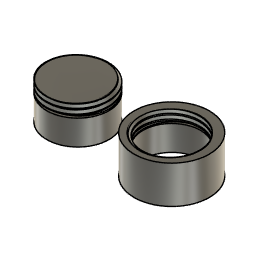
Threads Test (Autodesk Fusion 360 design; units mm, degrees)
Autodesk Fusion 360 part; units mm, degrees
sketch "Sketch1" plane through (0, 0, 0) normal (0, 0, 1) x (1, 0, 0)
  circle A0 centre (0, 0) radius 25
  dimension "d1" = 50
  constraint coincident A0.centre origin
  measures "d1" diameter of A0
extrude "Extrude1" add sketch "Sketch1" along normal blind 30 makes body 1
thread "Thread1" "ISO Metric profile 50.0 M50x4 6g" major diameter 49.7025 minor diameter 45.1258 pitch 4 angle 60 modelled right hand crest width 0.569 on face at (24.8758, -2.4892, 20) from (0, 0, 20) to (0, 0, 30) crest through (24.8513, 0, -1) on bodies 1
sketch "Sketch2" plane through (0, 0, 0) normal (0, 0, 1) x (1, 0, 0)
  circle A0 centre (75, 0) radius 25
  circle A1 centre (75, 0) radius 30
  constraint concentric A0 A1
extrude "Extrude2" add sketch "Sketch2" along normal blind 30 separate body makes body 2
thread "Thread2" "ISO Metric profile 50.0 M50x4 6H" major diameter 50.4462 minor diameter 45.9699 pitch 4 angle 60 modelled right hand crest width 1.0823 on face at (99.8758, -2.4892, 20) from (75, 0, 20) to (75, 0, 30) crest through (97.9849, 0, 1) on bodies 2
